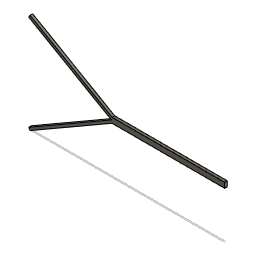
y_junction (Autodesk Fusion 360 design; units mm, degrees)
Autodesk Fusion 360 part; units mm, degrees
sketch "Sketch1" plane through (0, 0, 0) normal (0, 0, 1) x (1, 0, 0)
  line L0 (0.05, 3.8366) -> (6.5452, 0.0866)
  line L1 (6.5452, 0.0866) -> (6.4452, -0.0866)
  line L2 (6.4452, -0.0866) -> (-0.05, 3.6634)
  line L3 (-0.05, 3.6634) -> (0.05, 3.8366)
  line L4 (0, 0) -> (25, 0) construction
  line L5 (0.05, -3.8366) -> (6.5452, -0.0866)
  line L6 (-0.05, -3.6634) -> (0.05, -3.8366)
  line L7 (6.4452, 0.0866) -> (-0.05, -3.6634)
  line L8 (6.5452, -0.0866) -> (6.4452, 0.0866)
  line L9 (6.2952, 0.2) -> (15, 0.2)
  line L10 (15, 0.2) -> (15, -0.2)
  line L11 (15, -0.2) -> (6.2952, -0.2)
  line L12 (6.2952, -0.2) -> (6.2952, 0.2)
  line L13 (0, -3.75) -> (0, 3.75) construction
  point P0 (0, 3.75)
  point P1 (0, -3.75)
  point P2 (6.4952, 0)
  point P3 (6.2952, 0)
  dimension "d39" = 25
  dimension "d40" = 0.2
  dimension "d41" = 30
  dimension "d42" = 0.4
  dimension "d46" = 15
  dimension "d48" = 7.5
  constraint midpoint P0 L3
  constraint midpoint P2 L1
  constraint coincident L4.start origin
  constraint coincident P2 L4
  constraint parallel L0 L2
  constraint parallel L1 L3
  constraint perpendicular L0 L3
  constraint symmetric L0.start L4 L5.start
  constraint symmetric L0.end L4 L5.end
  constraint symmetric L1.end L4 L7.start
  constraint symmetric L2.end L4 L6.start
  constraint horizontal L9
  constraint vertical L10
  constraint horizontal L11
  constraint vertical L12
  constraint coincident L2 P3
  constraint coincident L7 P3
  constraint midpoint L12 P3
  constraint midpoint P1 L6
  constraint coincident P1 L13.start
  constraint coincident P0 L13.end
  constraint vertical L13
  constraint coincident L4.start L13
  measures "d39" distance of L4.start L4.end
  measures "d40" distance of L0 L2
  measures "d41" angle of L4 L7
  measures "d42" distance of L9.start L11.end
  measures "d46" distance of L10 L13
  measures "d48" distance of L5.start L5.end
extrude "Extrude1" add sketch "Sketch1" along normal blind 0.2
equation "d1001 = depth"
equation "channelwidth = 0.2 mm"
equation "depth = 0.2 mm"
equation "length = 15 mm"
equation "d40 = channelwidth"
equation "d41 = angle"
equation "d42 = channelwidth * 2"
equation "angle = 30 deg"
equation "d46 = length"
equation "d48 = length / 2"
